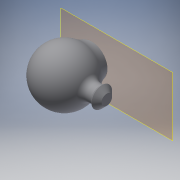
# Autodesk Inventor part: The Thing
Saved by Autodesk Inventor 2017 (Build 210142000, 142)
## iProperties
Created: 2017-03-09
Part Number: The Thing
Material: Generic
Document SubType Name: Modeling
Designer: PLTW
Density: 1 g/cm^3
Appearance: Default
Author: PLTW
Autodesk Inventor part; units mm, degrees
ref_plane "YZ Plane" through (0, 0, 0) normal (1, 0, 0) x (0, 1, 0)
ref_plane "XZ Plane" through (0, 0, 0) normal (0, 1, 0) x (-1, 0, 0)
sketch "Sketch3" plane through (0, 0, 0) normal (0, 0, 1) x (1, 0, 0)
  line L0 (-10.8841, 4.3559) -> (-10.16, 5.08)
  line L1 (-10.16, 5.08) -> (-7.62, 2.54)
  line L2 (-7.62, 2.54) -> (-7.62, -2.54)
  line L3 (-7.62, -2.54) -> (-10.16, -5.08)
  line L4 (-10.16, -5.08) -> (-10.8841, -4.3559)
  line L5 (-11.2504, 3.81) -> (-10.16, 4.9004)
  line L6 (-10.16, 4.9004) -> (-7.747, 2.4874)
  line L7 (-7.747, 2.4874) -> (-7.747, 0)
  line L8 (-7.747, 0) -> (-17.6004, 0)
  line L9 (-11.2504, 3.81) -> (-17.6004, 3.81)
  line L10 (-17.6004, 3.81) -> (-17.6004, 0)
  point P0 (0, 0)
  point P1 (-7.62, 0)
  dimension "d5" = 0.127
  dimension "d6" = 0.127
  dimension "d7" = 0.127
  dimension "d12" = 6.35
  dimension "d13" = 3.81
  constraints: 22 end point, 3 parallel, 3 perpendicular, 2 vertical, 1 horizontal, 1 horizontal alignment, 1 midpoint, 14 other
  measures "d5" distance between parallel lines of L0 L5
  measures "d6" distance between parallel lines of L1 L6
  measures "d7" distance between parallel lines of L2 L7
  measures "d12" distance of L5.start L9.end
  measures "d13" distance of L9.end L8.end
revolve "Revolution2" add sketch "Sketch3" angle 360 about axis through (-7.747, 0, 0) along (-1, 0, 0)
fillet "Fillet2" radius 0.127 3 edges at (-10.16, -4.9004, 0) (-11.2504, -3.81, 0) (-7.747, -2.4874, 0)
sketch "Sketch5" plane through (0, 0, 0) normal (0, 1, 0) x (-1, 0, 0)
  line L0 (17.6004, 3.81) -> (17.6004, -3.81) projected
  line L1 (17.6004, 3.81) -> (17.6004, -3.81) projected
  line L2 (11.303, 3.81) -> (11.303, -3.81) projected
  arc A0 (27.7604, 12.7) -> (27.7604, -12.7) centre (27.7604, 0) ccw
  line L3 (27.7604, 12.7) -> (27.7604, -12.7)
  point P0 (0, 0)
  dimension "d14" = 25.4
  dimension "d15" = 2.54
  constraints: 3 point on circle, 2 end point, 2 vertical alignment, 1 centre point, 1 horizontal alignment, 1 vertical
  measures "d14" distance of L3.end A0.start
  measures "d15" distance edge to line of A0 L0
revolve "Revolution3" add sketch "Sketch5" angle 360 about axis through (-27.7604, 0, 12.7) along (0, 0, -1)
ref_plane "Work Plane1" through (0, 0, -12.7) normal (0, 0, 1) x (1, 0, 0)
sketch "Sketch8" plane through (0, 0, -12.7) normal (0, 0, 1) x (1, 0, 0)
  line L0 (-15.6454, -3.81) -> (-15.6454, 3.81) projected
  circle A0 centre (-27.7622, 0) radius 7.62
  point P0 (0, 0)
  dimension "d18" = 27.7622
  dimension "d19" = 15.24
  constraints: 1 centre point, 1 coincident, 1 horizontal alignment
  measures "d18" distance of point (-27.762, 0) point (0, 0)
  measures "d19" diameter of A0
extrude "Extrusion1" add sketch "Sketch8" along normal up to next
fillet "Fillet3" radius 12.7 1 edges at (-35.3822, -0.0004, -10.1586)
fillet "Fillet4" radius 3.175 3 edges at (-15.6454, -3.81, 0) (-15.6454, 2.6939, 2.6943) (-15.6454, 2.6939, -2.6943)
equation "\"d6\" = d5"
equation "\"d7\" = d5"
body "Solid2"
